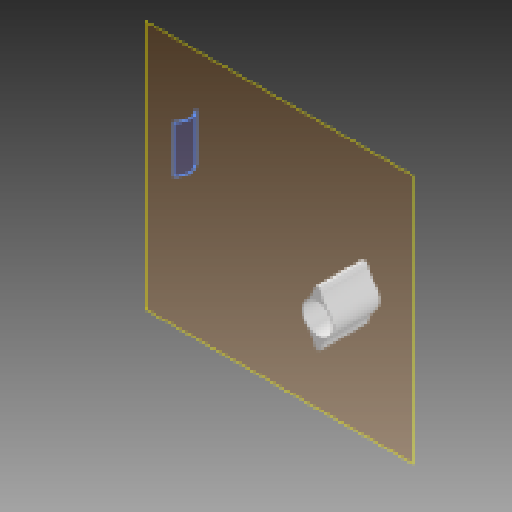
# Autodesk Inventor part: Крепление конденсатора
Saved by Autodesk Inventor 2023 (Build 270158000, 158)
## iProperties
Created: 2025-04-17
Part Number: Крепление конденсатора
Material: Типовые
Document SubType Name: Modeling
Designer: Ivan
Density: 1 g/cm^3
Appearance: По умолчанию
Author: Ivan
Autodesk Inventor part; units mm, degrees
ref_plane "XZ Plane" through (0, 0, 0) normal (0, 1, 0) x (-1, 0, 0)
ref_plane "XY Plane" through (0, 0, 0) normal (0, 0, 1) x (1, 0, 0)
ref_plane "РабПлоскость1" through (0, 0, 0) normal (0, 0, 1) x (1, 0, 0)
sketch "Эскиз1" plane through (0, 0, 0) normal (0, 0, 1) x (1, 0, 0)
  circle A0 centre (72.7898, 20) radius 1.5 construction
  circle A1 centre (72.7898, -20) radius 1.5 construction
  line L0 (72.7898, 20) -> (72.7898, -20) construction
  circle A2 centre (72.7898, 0) radius 13.6
  circle A3 centre (72.7898, 20) radius 3.5
  circle A4 centre (72.7898, -20) radius 3.5
  line L1 (76.2898, 20) -> (69.2898, 20) construction
  line L2 (76.2898, -20) -> (69.2898, -20) construction
  line L3 (82.4064, 9.6167) -> (63.1731, -9.6167) construction
  line L4 (82.4064, -9.6167) -> (63.1731, 9.6167) construction
  arc A5 (76.2898, 20) -> (82.4064, 9.6167) centre (99.4251, 26.6354) ccw
  arc A6 (63.1731, 9.6167) -> (69.2898, 20) centre (46.1544, 26.6354) ccw
  arc A7 (69.2898, -20) -> (63.1731, -9.6167) centre (46.1544, -26.6354) ccw
  arc A8 (82.4064, -9.6167) -> (76.2898, -20) centre (99.4251, -26.6354) ccw
  circle A9 centre (72.7898, 0) radius 12.6
  point P0 (0, 0)
  point P1 (72.7898, 0)
  dimension "d0" = 27.2
  dimension "d3" = 7
  dimension "d4" = 45
  dimension "d5" = 25.2
  constraints: 16 point on circle, 10 end point, 8 centre point, 8 coincident, 5 midpoint, 4 tangent, 2 horizontal, 1 equal radius, 1 perpendicular, 1 vertical
  measures "d0" diameter of A2
  measures "d3" diameter of A3
  measures "d4" angle of L4 L0
  measures "d5" diameter of A9
extrude "Выдавливание1" add sketch "Эскиз1" along normal blind 40
hole "Отверстие1" at (72.7898, 20, 0) at (72.7898, -20, 0) direction (0, 0, 1) diameter 3.8 depth 6
sketch "Эскиз2" plane through (0, 0, 0) normal (0, 1, 0) x (-1, 0, 0)
  point P0 (0, 0)
ref_plane "РабПлоскость2" through (72.7898, -23.5, 40) normal (1, 0, 0) x (0, 1, 0)
